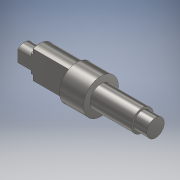
# Autodesk Inventor part: IP axle
Saved by Autodesk Inventor 2017 (Build 210142000, 142)
## iProperties
Created: 2018-07-24
Part Number: IP axle
Material: Stainless Steel
Document SubType Name: Modeling
Designer: jakub.tomczynski
Density: 8 g/cm^3
Appearance: Semi-Polished
Author: jakub.tomczynski
Autodesk Inventor part; units mm, degrees
ref_plane "YZ Plane" through (0, 0, 0) normal (1, 0, 0) x (0, 1, 0)
ref_plane "XZ Plane" through (0, 0, 0) normal (0, 1, 0) x (-1, 0, 0)
ref_plane "XY Plane" through (0, 0, 0) normal (0, 0, 1) x (1, 0, 0)
sketch "Sketch1" plane through (0, 0, 0) normal (0, 0, 1) x (1, 0, 0)
  line L0 (-7.5, 0) -> (7.5, 0)
  line L1 (-7.5, 0) -> (-7.5, 1)
  line L2 (-7.5, 1) -> (-6, 1)
  line L3 (-6, 1) -> (-6, 1.25)
  line L4 (-6, 1.25) -> (-5.75, 1.25)
  line L5 (-5.75, 1.25) -> (-5.75, 1.75)
  line L6 (1.25, 1.25) -> (6, 1.25)
  line L7 (6, 1.25) -> (6, 1)
  line L8 (6, 1) -> (7.5, 1)
  line L9 (7.5, 1) -> (7.5, 0)
  line L10 (0, 0) -> (0, -6.3915) construction
  line L11 (-5.75, 1.75) -> (-1.5, 1.75)
  line L12 (-1.5, 1.75) -> (-1.5, 2)
  line L13 (-1.5, 2) -> (1.25, 2)
  line L14 (1.25, 2) -> (1.25, 1.25)
  dimension "d0" = 15
  dimension "d1" = 1.5
  dimension "d2" = 2
  dimension "d3" = 2.5
  dimension "d8" = 0.25
  dimension "d9" = 3.5
  dimension "d10" = 4
  dimension "d11" = 4.25
  dimension "d12" = 6.25
  constraints: 32 end point, 9 perpendicular, 4 point on line, 2 horizontal, 2 vertical, 1 midpoint, 2 other
  measures "d0" distance between parallel lines of L9 L1
  measures "d1" distance between parallel lines of L3 L1
  measures "d2" diameter of L2 L0
  measures "d3" diameter of L4 L0
  measures "d8" distance between parallel lines of L5 L3
  measures "d9" diameter of L11 L0
  measures "d10" diameter of L13 L0
  measures "d11" distance between parallel lines of L12 L5
  measures "d12" distance between parallel lines of L9 L14
revolve "Revolution1" add sketch "Sketch1" angle 360 about axis through (-7.5, 0, 0) along (1, 0, 0)
sketch "Sketch2" plane through (-7.5, 0, 0) normal (-1, 0, 0) x (0, 0, 1)
  circle A0 centre (0, 0) radius 2 projected
  line L0 (-1.854, -0.75) -> (1.854, -0.75)
  point P0 (0, 0)
  dimension "d13" = 0.75
  constraints: 2 end point, 2 point on circle, 1 horizontal
  measures "d13" distance from line of point (0, 0) L0
extrude "Extrusion1" cut sketch "Sketch2" against normal up to surface (6 mm away) contours L0 A0 picked at (0, -1.1667)
body "Solid1"
